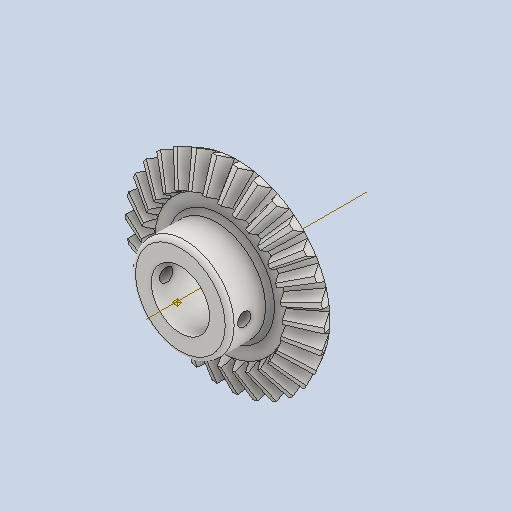
# Autodesk Inventor part: NagyKupkerek
Saved by Autodesk Inventor 2023.3 (Build 273359000, 359)
## iProperties
CustomPartVersion: 1
Created: 2023-11-24
Part Number: NagyKupkerek
Material: Steel, Mild
Document SubType Name: Modeling
Designer: Csábi-Kis Henrik
Categories: <?xml version="1.0" encoding="UTF-16"?> <MemberInstance><Categories><FamilyTemplate><FamilyTemplateParameter ValueType="xs:double" Id="1" ObjectReferenceKey="da_z" ObjectType="kUserParameterObject"/><FamilyTemplateParameter ValueType="xs:double" Id="2" ObjectReferenceKey="da_b" ObjectType="kUserParameterObject"/><FamilyTemplateParameter ValueType="xs:double" Id="3" ObjectReferenceKey="da_beta" ObjectType="kUserParameterObject"/><FamilyTemplateParameter ValueType="xs:double" Id="4" ObjectReferenceKey="da_dae" ObjectType="kUserParameterObject"/><FamilyTemplateParameter ValueType="xs:double" Id="5" ObjectReferenceKey="da_ve" ObjectType="kUserParameterObject"/><FamilyTemplateParameter ValueType="xs:double" Id="6" ObjectReferenceKey="da_omega" ObjectType="kUserParameterObject"/><FamilyTemplateParameter ValueType="xs:string" Id="7" ObjectReferenceKey="EAIAABAAAAAAHwAAAAAAAIAAAAAAAAAA" ObjectType="83914240" SubObjectId="SurfaceGeometry"/></FamilyTemplate><ParamToTemplateMap><ParamToTemplate CategoryParameter="//CategoryParameter[@InternalName='046C89C9-8512-4d59-83FE-43B91F4F132A']" TemplateParameter="1"/><ParamToTemplate CategoryParameter="//CategoryParameter[@InternalName='2552DF32-E462-4b46-AEBF-C6C7768E72AC']" TemplateParameter="2"/><ParamToTemplate CategoryParameter="//CategoryParameter[@InternalName='C9EE641D-15FC-4fae-A226-E94C4372FDD7']" TemplateParameter="3"/><ParamToTemplate><ParamToTemplate CategoryParameter="//CategoryParameter[@InternalName='00B6519A-459B-49c7-AD84-2E56D39A5744']" ConstantValue="0.000000"/></ParamToTemplate><ParamToTemplate><ParamToTemplate CategoryParameter="//CategoryParameter[@InternalName='04B31F0E-C7A6-4894-AA32-9629BEFACF47']" ConstantValue="1.000000"/></ParamToTemplate><ParamToTemplate><ParamToTemplate CategoryParameter="//CategoryParameter[@InternalName='43CBEC2E-7847-49e7-A936-2F7889FCB2D9']" ConstantValue="0.200000"/></ParamToTemplate><ParamToTemplate><ParamToTemplate CategoryParameter="//CategoryParameter[@InternalName='B1EFC894-105D-4ebd-86BF-FA20ED196853']" ConstantValue="0.300000"/></ParamToTemplate><ParamToTemplate><ParamToTemplate CategoryParameter="//CategoryParameter[@InternalName='51175063-3D10-4879-93E8-6246FE8B403D']" ConstantValue="2060000000.000000"/></ParamToTemplate><ParamToTemplate><ParamToTemplate CategoryParameter="//CategoryParameter[@InternalName='A3A52E27-4454-46a9-B0BD-C932399B70AF']" ConstantValue="0.300000"/></ParamToTemplate><ParamToTemplate CategoryParameter="//CategoryParameter[@InternalName='2A200944-5A8C-41ca-B96E-8520D2E510F1']" TemplateParameter="4"/><ParamToTemplate><ParamToTemplate CategoryParameter="//CategoryParameter[@InternalName='1A637F62-92C8-44bc-B81F-10802510B579']" ConstantValue="3.150540"/></ParamToTemplate><ParamToTemplate CategoryParameter="//CategoryParameter[@InternalName='B52DD4BE-6863-48fb-BF58-89EF6F9EC65C']" TemplateParameter="5"/><ParamToTemplate><ParamToTemplate CategoryParameter="//CategoryParameter[@InternalName='3956BFF2-84D2-457d-93C2-9B0613DEBA67']" ConstantValue="0.724744"/></ParamToTemplate><ParamToTemplate CategoryParameter="//CategoryParameter[@InternalName='739CFA02-461B-4bf8-8049-181FCAD8B28F']" TemplateParameter="6"/><ParamToTemplate><ParamToTemplate CategoryParameter="//CategoryParameter[@InternalName='A27E999F-E2CE-4481-8A2A-EBF499C4C3C5']" ConstantValue="0.000000"/></ParamToTemplate><ParamToTemplate><ParamToTemplate CategoryParameter="//CategoryParameter[@InternalName='9E1B4470-B2D3-4ff1-B813-535BB4CDF51A']" ConstantValue="3520000.000000"/></ParamToTemplate><ParamToTemplate><ParamToTemplate CategoryParameter="//CategoryParameter[@InternalName='F8452263-BFF6-458c-9FB1-07C4B99E95CD']" ConstantValue="11400000.000000"/></ParamToTemplate><ParamToTemplate><ParamToTemplate CategoryParameter="//CategoryParameter[@InternalName='3E3BB259-FD49-497f-8171-6EBC954A3479']" ConstantValue="2.000000"/></ParamToTemplate><ParamToTemplate CategoryParameter="//CategoryParameter[@InternalName='27C3BAF2-7550-4e4b-AE2C-0DB134B7D9B7']" TemplateParameter="7"/></ParamToTemplateMap><Category DisplayName="Gear" InternalName="DC85795E-93AB-48d5-8EEE-5A27447B64BD" Mnemonic="Gear"><CategoryParameter DisplayName="z" InternalName="046C89C9-8512-4d59-83FE-43B91F4F132A" Mnemonic="z"/><CategoryParameter DisplayName="b" InternalName="2552DF32-E462-4b46-AEBF-C6C7768E72AC" Mnemonic="b"/><CategoryParameter DisplayName="||b|" InternalName="C9EE641D-15FC-4fae-A226-E94C4372FDD7" Mnemonic="beta"/><CategoryParameter DisplayName="x" InternalName="00B6519A-459B-49c7-AD84-2E56D39A5744" Mnemonic="x"/><CategoryParameter DisplayName="a*" InternalName="04B31F0E-C7A6-4894-AA32-9629BEFACF47" Mnemonic="a"/><CategoryParameter DisplayName="c*" InternalName="43CBEC2E-7847-49e7-A936-2F7889FCB2D9" Mnemonic="c"/><CategoryParameter DisplayName="r|.f|*" InternalName="B1EFC894-105D-4ebd-86BF-FA20ED196853" Mnemonic="rf"/><CategoryParameter DisplayName="E" InternalName="51175063-3D10-4879-93E8-6246FE8B403D" Mnemonic="E"/><CategoryParameter DisplayName="||m|" InternalName="A3A52E27-4454-46a9-B0BD-C932399B70AF" Mnemonic="mi"/><Category DisplayName="BevelGear" InternalName="0C98F69A-0C2B-4791-B2FE-7691BB227E77" Mnemonic="BevelGear"><CategoryParameter DisplayName="d|.ae|" InternalName="2A200944-5A8C-41ca-B96E-8520D2E510F1" Mnemonic="dae"/><CategoryParameter DisplayName="d|.ai|" InternalName="1A637F62-92C8-44bc-B81F-10802510B579" Mnemonic="dai"/><CategoryParameter DisplayName="A|.e|" InternalName="B52DD4BE-6863-48fb-BF58-89EF6F9EC65C" Mnemonic="ve"/><CategoryParameter DisplayName="A|.i|" InternalName="3956BFF2-84D2-457d-93C2-9B0613DEBA67" Mnemonic="vi"/><CategoryParameter DisplayName="||S|" InternalName="739CFA02-461B-4bf8-8049-181FCAD8B28F" Mnemonic="omega"/><CategoryParameter DisplayName="x|.t|" InternalName="A27E999F-E2CE-4481-8A2A-EBF499C4C3C5" Mnemonic="xt"/><CategoryParameter DisplayName="||s||.Flim|" InternalName="9E1B4470-B2D3-4ff1-B813-535BB4CDF51A" Mnemonic="sFlim"/><CategoryParameter DisplayName="||s||.Hlim|" InternalName="F8452263-BFF6-458c-9FB1-07C4B99E95CD" Mnemonic="sHlim"/><CategoryParameter DisplayName="type" InternalName="3E3BB259-FD49-497f-8171-6EBC954A3479" Mnemonic="type"/><CategoryParameter DisplayName="PitchDiameter" InternalName="27C3BAF2-7550-4e4b-AE2C-0DB134B7D9B7" Mnemonic="IDS_PITCHDIAM"/></Category></Category></Categories></MemberInstance>
Mass: 50.7421 g
Surface Area: 48.2492 cm^2
Volume: 6.46396 cm^3
Density: 7.85 g/cm^3
Appearance: Steel
Author: Csábi-Kis Henrik
Autodesk Inventor part; units mm, degrees
ref_plane "Mesh Plane2" through (0, 0, 0) normal (0.9945219, 0.1045285, 0) x (0, 0, 1)
sketch "Teeth Body Sketch" plane through (0, 0, 0) normal (1, 0, 0) x (0, 1, 0)
  line L0 (0, 0) -> (20.6425, -12.9541) construction
  line L1 (20.6425, -12.9541) -> (22.1229, -10.1782)
  line L2 (22.1229, -10.1782) -> (0, 0) construction
  line L3 (21.45, -11.44) -> (0, 0) construction
  line L4 (14.6985, -9.224) -> (15.7527, -7.2474)
  line L5 (20.6425, -12.9541) -> (14.6985, -9.224)
  line L6 (22.1229, -10.1782) -> (15.7527, -7.2474)
  line L7 (0, -15.5449) -> (0, 2.5908) projected
  line L8 (0, -11.44) -> (22.1229, -11.44) construction
  dimension "d0" = 42.9
  dimension "d1" = 41.2849
  dimension "d2" = 44.2459
  dimension "d3" = 7
  dimension "d4" = 10.1782
  constraints: 16 end point, 4 point on line, 3 perpendicular, 2 collinear, 1 horizontal alignment, 1 vertical alignment
  measures "d0" diameter of L3.start L7
  measures "d1" diameter of L0.end L7
  measures "d2" diameter of L1.end L7
  measures "d3" distance between parallel lines of L1 L4
  measures "d4" vertical distance of L1.end L0.start
revolve "Teeth Body" add sketch "Teeth Body Sketch" angle 360 about axis through (0, 0, 0) along (0, 0, 1)
ref_plane "Tooth Plane" through (0, 21.45, -11.44) normal (0, -0.8823529, 0.4705882) x (1, 0, 0)
sketch "Start Sketch" plane through (0, 21.45, -11.44) normal (0, -0.8823529, 0.4705882) x (1, 0, 0)
  line L0 (0, -55.1747) -> (0, 11.9796) projected
  arc A0 (-0.4945, -2.0935) -> (-2.2555, 2.3207) centre (-16.1507, -5.7809) ccw
  arc A1 (2.2555, 2.3207) -> (0.4945, -2.0935) centre (16.1507, -5.7809) ccw
  line L1 (-0.4945, -2.0935) -> (0.4945, -2.0935)
  arc A2 (2.2555, 2.3207) -> (-2.2555, 2.3207) centre (0, -45.5812) ccw
  dimension "d7" = 16.0845
  dimension "d8" = 16.1507
  dimension "d9" = 39.8004
  dimension "d57" = 47.955
  dimension "d58" = 43.4877
  constraints: 6 point on circle, 3 centre point, 3 symmetric about line, 2 end point, 1 coincident, 1 perpendicular, 1 other
  measures "d7" radius of A0
  measures "d8" horizontal distance of point (0, -45.581) A0.centre
  measures "d9" vertical distance of point (0, -45.581) A0.centre
  measures "d57" radius of A2
  measures "d58" distance from line of A2.centre L1
sketch "End Sketch" plane through (0, 15.1347, -8.0719) normal (0, -0.8823529, 0.4705882) x (1, 0, 0)
  line L0 (0, -36.6607) -> (0, 7.9598) projected
  arc A0 (-0.3489, -1.4772) -> (-1.5915, 1.6375) centre (-11.3956, -4.0789) ccw
  arc A1 (1.5915, 1.6375) -> (0.3489, -1.4772) centre (11.3956, -4.0789) ccw
  line L1 (-0.3489, -1.4772) -> (0.3489, -1.4772)
  arc A2 (1.5915, 1.6375) -> (-1.5915, 1.6375) centre (0, -32.1613) ccw
  dimension "d12" = 11.349
  dimension "d15" = 11.3956
  dimension "d16" = 28.0824
  dimension "d59" = 33.8362
  dimension "d60" = 30.6842
  constraints: 6 point on circle, 3 centre point, 3 symmetric about line, 2 end point, 1 coincident, 1 other
  measures "d12" radius of A0
  measures "d15" horizontal distance of A0.centre point (0, -32.161)
  measures "d16" vertical distance of A0.centre point (0, -32.161)
  measures "d59" radius of A2
  measures "d60" distance from line of A2.centre L1
loft "Loft" cut profiles "Start Sketch", "End Sketch"
pattern_circular "Circular Pattern" count 30 over 360 about axis through (0, 0, 0) along (0, 0, 1) of "Loft"
ref_plane "End Plane" through (0, 15.1347, -8.0719) normal (0, -0.8823529, 0.4705882) x (1, 0, 0)
sketch3d "3D Sketch Right"
ref_plane "End Plane Right" through (-2.4578, 14.9338, -8.0719) normal (0.1432877, -0.8706408, 0.4705882) x (0.9867262, 0.1623927, 0)
sketch "End Sketch Right" plane through (-2.4578, 14.9338, -8.0719) normal (0.1432877, -0.8706408, 0.4705882) x (0.9867262, 0.1623927, 0)
  arc A0 (-0.3489, -1.4772) -> (-1.5915, 1.6375) centre (-11.3956, -4.0789) ccw
  line L0 (0, -41.1764) -> (0, 10.6006) projected
  arc A1 (1.5915, 1.6375) -> (0.3489, -1.4772) centre (11.3956, -4.0789) ccw
  line L1 (-0.3489, -1.4772) -> (0.3489, -1.4772)
  arc A2 (1.5915, 1.6375) -> (-1.5915, 1.6375) centre (0, -32.1613) ccw
  dimension "d70" = 11.3956
  dimension "d71" = 28.0824
  dimension "d72" = 11.349
  dimension "d73" = 30.6842
  dimension "d74" = 33.8362
  constraints: 6 point on circle, 3 centre point, 3 symmetric about line, 2 end point, 1 coincident, 1 perpendicular, 1 other
  measures "d70" horizontal distance of A2.centre A0.centre
  measures "d71" vertical distance of point (0, -32.161) A0.centre
  measures "d72" radius of A0
  measures "d73" distance from line of point (0, -32.161) L1
  measures "d74" radius of A2
feature "Loft Right" [suppressed]
pattern_circular "Circular Pattern Right" [suppressed]
sketch3d "3D Sketch Left"
ref_plane "End Plane Left" through (2.5171, 14.9338, -8.116) normal (-0.1464952, -0.8691517, 0.47235) x (0.9860912, -0.1662053, 0)
sketch "End Sketch Left" plane through (2.5171, 14.9338, -8.116) normal (-0.1464952, -0.8691517, 0.47235) x (0.9860912, -0.1662053, 0)
  line L0 (0, -42.093) -> (0, 11.5824) projected
  arc A0 (-0.3489, -1.4428) -> (-1.5915, 1.6718) centre (-11.3956, -4.0446) ccw
  arc A1 (1.5915, 1.6718) -> (0.3489, -1.4428) centre (11.3956, -4.0446) ccw
  line L1 (-0.3489, -1.4428) -> (0.3489, -1.4428)
  ellipse E0 centre (0, -6.388) end of major axis (15.7527, -6.388) minor radius 7.4408 projected
  arc A2 (1.5915, 1.6718) -> (-1.5915, 1.6718) centre (0, -32.127) ccw
  dimension "d56" = 7.4408
  dimension "d30" = 11.349
  dimension "d31" = 11.3956
  dimension "d32" = 28.0824
  dimension "d61" = 33.8362
  dimension "d62" = 30.6842
  constraints: 6 point on circle, 3 centre point, 3 symmetric about line, 2 end point, 1 coincident, 2 other
  measures "d30" radius of A0
  measures "d31" horizontal distance of point (0, -32.127) A0.centre
  measures "d32" vertical distance of A0.centre point (0, -32.127)
  measures "d61" radius of A2
  measures "d62" distance from line of point (0, -32.127) L1
feature "Loft Left" [suppressed]
pattern_circular "Circular Pattern Left" [suppressed]
sketch "Body Sketch" plane through (0, 0, 0) normal (1, 0, 0) x (0, 1, 0)
  line L0 (0, -13.8067) -> (0, -7.8385) projected
  line L1 (20.6425, -12.9541) -> (14.6985, -9.224) projected
  line L2 (14.6985, -9.224) -> (0, -9.224)
  line L3 (20.6425, -12.9541) -> (0, -12.9541)
  constraints: 4 end point, 2 perpendicular, 2 point on line
revolve "Fix Body" add sketch "Body Sketch" angle 360 about axis through (0, 0, 0) along (0, 0, 1)
sketch "Sketch6" plane through (0, 0, 0) normal (1, 0, 0) x (0, 1, 0)
  line L0 (21.45, -11.44) -> (0, 0) projected
  line L1 (0, -13.728) -> (0, 2.288) projected
surface revolve "Pitch Diameter" sketch "Sketch6" angle 360 about axis through (0, 0, 0) along (0, 0, 1) shown no curves L0
sketch "Sketch8" plane through (0, 0, -9.224) normal (0, 0, 1) x (1, 0, 0)
  circle A0 centre (0, 0) radius 11
  dimension "d94" = 22
  constraints: 1 centre point, 1 coincident
  measures "d94" diameter of A0
extrude "Extrusion1" add sketch "Sketch8" along normal blind 9
sketch "Sketch9" plane through (0, 0, 0) normal (1, 0, 0) x (0, 1, 0)
  line L0 (-1.5731, -12.9541) -> (1.5731, -12.9541) projected
  line L1 (0, 1.1243) -> (0, -15.3136) projected
  point P0 (0, -3.5001)
  dimension "d97" = 9.454
  constraints: 1 point on line
  measures "d97" distance from line of L0 point (0, -3.5)
sketch "Sketch10" plane through (0, 0, -0.224) normal (0, 0, 1) x (1, 0, 0)
  point P0 (0, 0)
hole "Hole1" at (0, 0, -0.224) direction (0, 0, -1) diameter 13 end through all
hole "Hole2" at (0, 0, -3.5001) direction (-1, 0, 0) diameter 3 end through all both
fillet "Fillet1" radius 1 2 edges at (-11, 0, -0.224) (-11, 0, -9.224)
equation "\"d0\" = da_de"
equation "\"d1\" = da_dfe"
equation "\"d2\" = da_dae"
equation "\"d3\" = da_b"
equation "\"d4\" = da_ve"
equation "\"d7\" = fd_rr"
equation "\"d8\" = fd_x"
equation "\"d9\" = fd_y"
equation "\"d57\" = 0.5 * fd_dva + 0.3 * da_he"
equation "\"d58\" = 0.5 * fd_dva - 1.12 * da_he"
equation "\"da_teethtype\" = 0"
equation "\"d98\" = KupkerekBelsoCsatlakozas"
equation "\"d105\" = SzegAtmero"
equation "\"da_b\" = 7"
equation "\"da_de\" = 42.9"
equation "\"da_dae\" = 44.24588"
equation "\"da_dfe\" = 41.28494"
equation "\"da_le\" = 24.31"
equation "\"da_omega\" = 90deg"
equation "\"da_beta\" = 0"
equation "\"da_delta\" = 61.927513deg"
equation "\"da_alpha\" = 20deg"
equation "\"da_he\" = 3.146"
equation "\"da_ve\" = 10.17824"
equation "\"da_zv\" = 63.75"
equation "\"fd_loft\" = da_b + 0.05 * da_he"
equation "\"fd_x\" = fd_x1 + fd_x2"
equation "\"fd_y\" = fd_y1 - fd_y2"
equation "\"fd_dd\" = fd_dva - 0.8 * da_he"
equation "\"da_dvw\" = 91.1625"
equation "\"d11\" = fd_loft"
equation "\"da_dm\" = 36.72353"
equation "\"da_x\" = 0"
equation "\"da_m\" = 1.43"
equation "\"d50\" = da_omega"
equation "\"fd_rr\" = 16.084522"
equation "\"fd_dva\" = 94.0225"
equation "\"KupkerekBelsoCsatlakozas\" = 13"
equation "\"SzegAtmero\" = 3"
equation "\"fd_x1\" = 1.135481"
equation "\"fd_x2\" = 15.015215"
equation "\"fd_y1\" = 45.567105"
equation "\"fd_y2\" = 5.766731"
body "Solid1"
body "Srf1"
